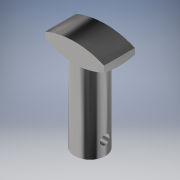
# Autodesk Inventor part: Stem
Saved by Autodesk Inventor 2018 (Build 220112000, 112)
## iProperties
Shininess: 64.0
Length Units: 11269
Angle Units: 11279
Time Units: 11290
Mass Units: 11283
Length Display Precision: 3
Angle Display Precision: 2
Compacted: True
Part Number: Stem
Document SubType Name: Modeling
Created: 2003-04-24
Designer: James M. Leake
Material: Steel, Mild
Density: 7.85 g/cm^3
Appearance: Semi-Polished
Density: 0.0
Volumn: 0.0
Area: 0.0
PropertySet Name: Model Information
Control State: 0
Master: False
Checked Out: False
Author: James M. Leake
Autodesk Inventor part; units mm, degrees
ref_plane "YZ Plane" through (0, 0, 0) normal (1, 0, 0) x (0, 1, 0)
sketch "Sketch1" plane through (0, 0, 0) normal (0, 0, 1) x (1, 0, 0)
  line L0 (-16.45, 0) -> (38.85, 0) projected
  line L1 (0, -84.7) -> (0, 23.1) projected
  line L2 (-12.5, -29.4576) -> (-12.5, -21.4576)
  line L3 (-12.5, -21.4576) -> (12.5, -21.4576)
  line L4 (12.5, -21.4576) -> (12.5, -29.4576)
  arc A0 (-12.5, -29.4576) -> (12.5, -29.4576) centre (0, 0) ccw
  arc A1 (0, -77) -> (0, -23) centre (0, -50) ccw
  line L5 (0, -77) -> (0, -23)
  dimension "d0" = 32
  dimension "d1" = 8
  dimension "d2" = 25
  dimension "d5" = 27
  dimension "d6" = 50
  constraints: 8 end point, 4 point on circle, 3 parallel, 2 centre point, 2 point on line, 1 coincident, 1 collinear, 1 perpendicular, 1 other
  measures "d0" radius of A0
  measures "d1" distance of L3.end L4.end
  measures "d2" distance of L2.end L3.end
  measures "d5" radius of A1
  measures "d6" distance from line of L0 A1.centre
extrude "Extrusion1" add sketch "Sketch1" along normal mid plane 13 contours A0 L2 L3 L1 | L1 A1 L4 A0 | A1 L1 L3 L4 picked at (1.4378, -26.1156)
revolve "Revolution1" cut sketch "Sketch1" angle 360 about axis through (0, -10, 0) along (0, 1, 0) keep common part contours L1 A0 L4 A1 | L1 A1 L4 A0
ref_plane "Work Plane1" through (0, -32, 0) normal (0, 1, 0) x (-1, 0, 0)
ref_plane "Work Plane2" through (0, 10, 0) normal (0, 1, 0) x (-1, 0, 0)
sketch "Sketch2" plane through (0, 10, 0) normal (0, 1, 0) x (-1, 0, 0)
  circle A0 centre (0, 0) radius 6.5
  line L0 (-12.5, 6.5) -> (12.5, 6.5) projected
  constraints: 1 centre point, 1 coincident, 1 tangent
extrude "Extrusion2" add sketch "Sketch2" against normal up to next
sketch "Sketch3" plane through (0, 0, 0) normal (1, 0, 0) x (0, 1, 0)
  line L0 (1.2, 0) -> (12.4, 0) projected
  circle A0 centre (4, 0) radius 2
  line L1 (10, 6.5) -> (10, -6.5) projected
  dimension "d11" = 4
  dimension "d12" = 6
  constraints: 1 centre point, 1 point on line
  measures "d11" diameter of A0
  measures "d12" distance from line of L1 A0.centre
extrude "Extrusion3" cut sketch "Sketch3" along normal through all both and the other way through all
body "Solid1"
